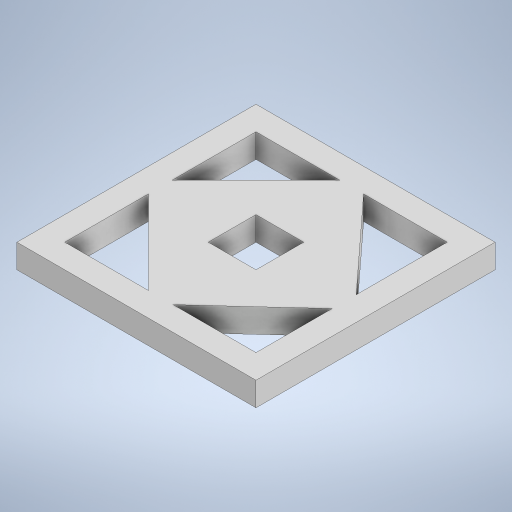
# Autodesk Inventor part: Panel
Saved by Autodesk Inventor 2023 (Build 270158000, 158)
## iProperties
Created: 2024-02-21
Part Number: Panel
Material: Generic
Document SubType Name: Modeling
Designer: tyler
Density: 1 g/cm^3
Appearance: Default
Author: tyler
Autodesk Inventor part; units mm, degrees
ref_plane "YZ Plane" through (0, 0, 0) normal (1, 0, 0) x (0, 1, 0)
ref_plane "XZ Plane" through (0, 0, 0) normal (0, 1, 0) x (-1, 0, 0)
ref_plane "XY Plane" through (0, 0, 0) normal (0, 0, 1) x (1, 0, 0)
sketch "Sketch1" plane through (0, 0, 0) normal (0, 1, 0) x (-1, 0, 0)
  line L0 (0, 0) -> (-254, 0)
  line L1 (-254, 0) -> (-254, -254)
  line L2 (-254, -254) -> (0, -254)
  line L3 (0, -254) -> (0, 0)
  line L4 (-25.4, -228.6) -> (-228.6, -228.6)
  line L5 (-228.6, -228.6) -> (-228.6, -25.4)
  line L6 (-228.6, -25.4) -> (-25.4, -25.4)
  line L7 (-25.4, -25.4) -> (-25.4, -228.6)
  line L8 (-25.4, -139.7) -> (-114.3, -228.6)
  line L9 (-25.4, -114.3) -> (-114.3, -25.4)
  line L10 (-139.7, -228.6) -> (-228.6, -131.82)
  line L11 (-228.6, -106.42) -> (-140.3985, -25.4)
  line L12 (-101.6, -152.4) -> (-152.4, -152.4)
  line L13 (-152.4, -152.4) -> (-152.4, -101.6)
  line L14 (-152.4, -101.6) -> (-101.6, -101.6)
  line L15 (-101.6, -101.6) -> (-101.6, -152.4)
  point P0 (-127, -25.4)
  point P1 (-127, -152.4)
  dimension "d0" = 254
  dimension "d1" = 254
  dimension "d2" = 203.2
  dimension "d3" = 203.2
  dimension "d4" = 25.4
  dimension "d7" = 88.9
  dimension "d8" = 88.9
  dimension "d9" = 88.9
  dimension "d10" = 88.9
  dimension "d15" = 50.8
  dimension "d16" = 50.8
  dimension "d17" = 76.2
  dimension "d18" = 76.2
  constraints: 32 end point, 8 point on line, 6 parallel, 4 perpendicular, 3 horizontal, 2 midpoint
  measures "d0" distance of L2.end L1.end
  measures "d1" distance of L1.end L0.end
  measures "d2" distance of L5.end L6.end
  measures "d3" distance of L4.end L5.end
  measures "d4" distance between parallel lines of L2 L4
  measures "d7" distance from line of L4 L8.start
  measures "d8" distance from line of L7 L8.end
  measures "d9" distance from line of L6 L9.start
  measures "d10" distance of L9.end L6.end
  measures "d15" distance of L13.end L14.end
  measures "d16" distance of L12.end L13.end
  measures "d17" distance between parallel lines of L5 L13
  measures "d18" distance from line of L4 point (-127, -152.4)
extrude "Extrusion1" add sketch "Sketch1" along normal blind 25.4 contours L3 L2 L1 L0 | L4 L10 L5 L11 L6 L9 L7 L8
body "Solid1"
